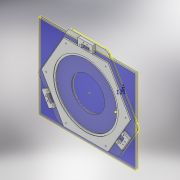
# Autodesk Inventor part: Bett Monster
Saved by Autodesk Inventor 2019 (Build 230136000, 136)
## iProperties
Created: 2018-08-03
Part Number: Bett Monster
Material: Generisch
Document SubType Name: Modeling
Designer: rene
Density: 1 g/cm^3
Appearance: Vorgabe
Author: rene
Autodesk Inventor part; units mm, degrees
ref_plane "YZ Plane" through (0, 0, 0) normal (1, 0, 0) x (0, 1, 0)
ref_plane "XZ Plane" through (0, 0, 0) normal (0, 1, 0) x (-1, 0, 0)
ref_plane "XY Plane" through (0, 0, 0) normal (0, 0, 1) x (1, 0, 0)
sketch "Bett" plane through (0, 0, 0) normal (0, 0, 1) x (1, 0, 0)
  circle A0 centre (0, 0) radius 175
  circle A1 centre (107.4996, -186.1957) radius 2.5
  line L0 (119.9996, -207.8464) -> (107.4996, -186.1957)
  line L1 (119.9996, -207.8465) -> (-120.0005, -207.8459)
  circle A2 centre (-107.5004, -186.1953) radius 2.5
  line L2 (-120.0004, -207.8459) -> (-107.5004, -186.1953)
  line L3 (-240.0001, 0.0004) -> (-120.0005, -207.8459)
  circle A3 centre (107.5004, 186.1953) radius 2.5
  line L4 (-119.9995, 207.8464) -> (120.0006, 207.8458)
  circle A4 centre (215.0001, -0.0004) radius 2.5
  line L5 (120.0006, 207.8458) -> (240.0001, -0.0006)
  circle A5 centre (-215.0001, 0.0004) radius 2.5
  line L6 (-240.0001, 0.0004) -> (-215.0001, 0.0004)
  circle A6 centre (-107.4996, 186.1957) radius 2.5
  line L7 (-240.0001, 0.0004) -> (-119.9995, 207.8464)
  line L8 (240.0001, -0.0006) -> (119.9996, -207.8465)
  circle A7 centre (0, 0) radius 165
  dimension "d0" = 350
  dimension "d1" = 240
  dimension "d2" = 207.8462
  dimension "d3" = 207.8462
  dimension "d4" = 119.9995
  dimension "d5" = 25
  dimension "d6" = 5
  dimension "d7" = 25
  dimension "d8" = 5
  dimension "d9" = 25
  dimension "d10" = 5
  dimension "d11" = 5
  dimension "d12" = 5
  dimension "d13" = 5
  dimension "d14" = 330
  constraints: 18 end point, 8 centre point, 8 coincident, 1 horizontal
  measures "d0" diameter of A0
  measures "d1" distance of L7.start L1.end
  measures "d2" distance from line of point (0, 0) L3
  measures "d3" distance from line of point (0, 0) L5
  measures "d4" horizontal distance of L5.start L5.end
  measures "d5" distance of L7.start L6.end
  measures "d6" diameter of A5
  measures "d7" distance of L0.start L0.end
  measures "d8" diameter of A1
  measures "d9" distance of L2.start L2.end
  measures "d10" diameter of A2
  measures "d11" diameter of A4
  measures "d12" diameter of A3
  measures "d13" diameter of A6
  measures "d14" diameter of A7
extrude "Extrusion Bett" add sketch "Bett" against normal blind 6 contours L1 L3 L7 L4 L5 L8
ref_plane "Arbeitsebene1" through (0, 0, -6) normal (0, 0, -1) x (-1, 0, 0)
sketch "Bett Ring" plane through (0, 0, -6) normal (0, 0, -1) x (-1, 0, 0)
  circle A0 centre (0, 0) radius 165
  circle A1 centre (0, 0) radius 175
  dimension "d18" = 350
  dimension "d19" = 330
  constraints: 2 centre point, 2 coincident
  measures "d18" diameter of A1
  measures "d19" diameter of A0
extrude "Extrusion Bett Ring" add sketch "Bett Ring" against normal blind 4
ref_plane "Arbeitsebene2" through (0, 0, -12) normal (0, 0, -1) x (-1, 0, 0)
sketch "Füsse" plane through (0, 0, -12) normal (0, 0, -1) x (-1, 0, 0)
  circle A0 centre (-107.4996, 186.1957) radius 2.5
  circle A1 centre (-107.4996, 186.1957) radius 5
  circle A2 centre (107.5004, 186.1953) radius 2.5
  circle A3 centre (107.5004, 186.1953) radius 5
  circle A4 centre (215.0001, -0.0004) radius 2.5
  circle A5 centre (215.0001, -0.0004) radius 5
  circle A6 centre (-215.0001, 0.0004) radius 5
  circle A7 centre (107.4996, -186.1957) radius 2.5
  circle A8 centre (107.4996, -186.1957) radius 5
  circle A9 centre (-107.5004, -186.1953) radius 5
  circle A10 centre (-107.5004, -186.1953) radius 2.5
  line L0 (-240.0001, 0.0004) -> (-215.0001, 0.0004)
  circle A11 centre (-215.0001, 0.0004) radius 2.5
  point P0 (0, 0)
  point P1 (0, 0)
  point P2 (0, 0)
  point P3 (0, 0)
  point P4 (0, 0)
  point P5 (0, 0)
  point P6 (0, 0)
  point P7 (165, -216.5064)
  point P8 (-165, -216.5064)
  point P9 (0, 0)
  point P10 (0, 0)
  point P11 (0, 0)
  point P12 (0, 0)
  point P13 (0, 0)
  dimension "d42" = 5
  dimension "d24" = 5
  dimension "d25" = 5
  dimension "d26" = 5
  dimension "d27" = 5
  dimension "d28" = 5
  dimension "d29" = 5
  dimension "d30" = 10
  dimension "d31" = 10
  dimension "d32" = 10
  dimension "d33" = 10
  dimension "d34" = 10
  dimension "d35" = 10
  constraints: 16 coincident, 12 centre point, 2 end point, 1 horizontal
  measures "d24" diameter of A11
  measures "d25" diameter of A7
  measures "d26" diameter of A10
  measures "d27" diameter of A4
  measures "d28" diameter of A2
  measures "d29" diameter of A0
  measures "d30" diameter of A3
  measures "d31" diameter of A5
  measures "d32" diameter of A8
  measures "d33" diameter of A9
  measures "d34" diameter of A1
  measures "d35" diameter of A6
extrude "Extrusion3" add sketch "Füsse" against normal blind 6
ref_plane "Arbeitsebene3" through (0, 0, -21) normal (0, 0, -1) x (-1, 0, 0)
sketch "Bodenplatte" plane through (0, 0, -21) normal (0, 0, -1) x (-1, 0, 0)
  circle A0 centre (-161.25, 93.0978) radius 3
  line L0 (-107.4998, 186.1959) -> (-214.9999, 0.0003) construction
  line L1 (0, 0) -> (-220.0773, 127.0617) construction
  line L2 (-262.7831, -22.1411) -> (-112.217, 238.6473)
  line L3 (-105.0001, 251.1473) -> (165, -216.5064) construction
  line L4 (-165, -216.5064) -> (104.9999, 251.1473) construction
  circle A1 centre (0, 0) radius 90
  circle A2 centre (-214.9999, 0.0003) radius 2.5
  circle A3 centre (-107.4998, 186.1959) radius 2.5
  circle A4 centre (-0.0001, 211.1473) radius 3
  line L5 (-90.5663, 251.1473) -> (90.5662, 251.1473)
  arc A5 (112.2168, 238.6473) -> (90.5662, 251.1473) centre (90.5662, 226.1473) ccw
  circle A6 centre (0, -186.1955) radius 3
  line L6 (150.5662, -216.5064) -> (-150.5663, -216.5064)
  line L7 (-270, -34.6411) -> (269.9999, -34.6411) construction
  circle A7 centre (107.4996, -186.1957) radius 2.5
  arc A8 (150.5662, -216.5064) -> (172.2168, -204.0064) centre (150.5662, -191.5064) ccw
  circle A9 centre (182.8589, -105.5736) radius 3
  line L8 (172.2168, -204.0064) -> (262.783, -47.1411)
  arc A10 (-90.5663, 251.1473) -> (-112.217, 238.6473) centre (-90.5663, 226.1473) ccw
  circle A11 centre (215.0001, -0.0004) radius 2.5
  line L9 (112.2168, 238.6473) -> (262.783, -22.1411)
  circle A12 centre (107.5004, 186.1953) radius 2.5
  circle A13 centre (161.25, 93.0978) radius 3
  line L10 (0, 0) -> (254.1234, 0) construction
  line L11 (107.5004, 186.1953) -> (215.0001, -0.0004) construction
  arc A14 (262.783, -47.1411) -> (262.783, -22.1411) centre (241.1324, -34.6411) ccw
  circle A15 centre (-107.5004, -186.1953) radius 2.5
  arc A16 (-172.2169, -204.0064) -> (-150.5663, -216.5064) centre (-150.5663, -191.5064) ccw
  circle A17 centre (-182.8589, -105.5737) radius 3
  line L12 (-172.2169, -204.0064) -> (-262.7831, -47.1411)
  arc A18 (-262.7831, -22.1411) -> (-262.7831, -47.1411) centre (-241.1325, -34.6411) ccw
  line L13 (-290, 0) -> (-289.695, 0.5283)
  dimension "d39" = 210
  dimension "d40" = 330
  dimension "d41" = 180
  dimension "d42" = 5
  dimension "d43" = 5
  dimension "d44" = 5
  dimension "d45" = 5
  dimension "d46" = 5
  dimension "d47" = 6
  dimension "d48" = 6
  dimension "d49" = 6
  dimension "d50" = 150
  dimension "d51" = 6
  dimension "d52" = 6
  dimension "d53" = 6
  dimension "d54" = 5
  constraints: 28 end point, 19 centre point, 12 point on circle, 12 tangent, 10 coincident, 3 parallel, 2 horizontal, 1 equal length, 1 perpendicular, 1 point on line
  measures "d39" distance of L3.start L4.end
  measures "d40" distance of L3.end L4.start
  measures "d41" diameter of A1
  measures "d42" diameter of A2
  measures "d43" diameter of A7
  measures "d44" diameter of A15
  measures "d45" diameter of A11
  measures "d46" diameter of A12
  measures "d47" diameter of A4
  measures "d48" diameter of A17
  measures "d49" diameter of A9
  measures "d50" angle of L10 L1
  measures "d51" diameter of A6
  measures "d52" diameter of A0
  measures "d53" diameter of A13
  measures "d54" diameter of A3
extrude "Extrusion4" add sketch "Bodenplatte" against normal blind 9
sketch "Skizze5" plane through (0, 0, -12) normal (0, 0, -1) x (-1, 0, 0)
  line L0 (0.0004, 251.1474) -> (0.0004, 250.619)
  line L1 (0.0004, 250.619) -> (0.0004, 251.1474)
  line L2 (0.0004, 250.619) -> (0.0004, 251.1474)
  line L3 (0, 231.1474) -> (20.0002, 251.1474) construction
  line L4 (0, 231.1474) -> (20.0004, 231.1478)
  line L5 (20.0004, 231.1478) -> (0.0004, 251.1471) construction
  line L6 (40.0005, 211.1469) -> (40.0005, 251.1474)
  line L7 (-172.8592, -122.8938) -> (-190.1797, -132.8938)
  circle A0 centre (-176.5195, -136.554) radius 2.6
  line L8 (-172.8592, -122.8938) -> (-180.1797, -150.2143) construction
  line L9 (-162.8592, -140.2143) -> (-172.8592, -122.8938)
  line L10 (-162.8592, -140.2143) -> (-190.1797, -132.8938) construction
  line L11 (-197.5002, -160.2143) -> (-162.8592, -140.2143)
  line L12 (-210.1801, -98.2531) -> (-192.8588, -88.2526)
  circle A1 centre (-206.5195, -84.5926) radius 2.6
  line L13 (-202.8588, -70.932) -> (-192.8588, -88.2526)
  line L14 (-192.8588, -88.2526) -> (-220.1788, -80.9317) construction
  line L15 (-202.8588, -70.932) -> (-210.1801, -98.2531) construction
  line L16 (-202.8588, -70.932) -> (-237.5002, -90.9322)
  circle A2 centre (-204.2437, -129.1252) radius 2.6
  line L17 (-190.1797, -132.8938) -> (-200.1795, -115.5737)
  line L18 (-190.1797, -132.8938) -> (-217.5, -125.5732) construction
  line L19 (-200.1795, -115.5737) -> (-208.0747, -141.8989) construction
  line L20 (-217.5002, -125.5733) -> (-217.0427, -125.3091)
  line L21 (-217.0427, -125.3091) -> (-217.5002, -125.5733)
  line L22 (-217.0427, -125.3091) -> (-217.5002, -125.5733)
  circle A3 centre (-213.8398, -111.9133) radius 2.6
  line L23 (-237.5002, -90.9322) -> (-197.5002, -160.2143)
  line L24 (-200.1795, -115.5737) -> (-210.1801, -98.2531)
  line L25 (-210.1801, -98.2531) -> (-217.5, -125.5732) construction
  line L26 (-200.1795, -115.5737) -> (-227.5001, -108.253) construction
  line L27 (162.8584, -140.2149) -> (172.8584, -122.8943)
  line L28 (190.1797, -132.8947) -> (172.8584, -122.8943)
  circle A4 centre (176.519, -136.5548) radius 2.6
  line L29 (172.8584, -122.8943) -> (180.1783, -150.2146) construction
  line L30 (162.8584, -140.2149) -> (190.1797, -132.8947) construction
  line L31 (162.8584, -140.2149) -> (197.4998, -160.2151)
  circle A5 centre (203.8397, -129.234) radius 2.6
  line L32 (200.1795, -115.5737) -> (190.1797, -132.8947)
  line L33 (182.8584, -105.5739) -> (182.8586, -105.5735)
  line L34 (182.8586, -105.5735) -> (182.8584, -105.5739)
  line L35 (190.1797, -132.8947) -> (217.4995, -125.5739) construction
  line L36 (200.1795, -115.5737) -> (207.4999, -142.8944) construction
  line L37 (217.0422, -125.3099) -> (217.4998, -125.5741)
  line L38 (217.4998, -125.5741) -> (217.0422, -125.3099)
  line L39 (217.0422, -125.3099) -> (217.4998, -125.5741)
  circle A6 centre (213.9476, -112.3176) radius 2.6
  line L40 (197.4998, -160.2151) -> (237.4998, -90.9331)
  line L41 (210.1792, -98.2536) -> (200.1795, -115.5737)
  line L42 (210.1792, -98.2536) -> (217.4995, -125.5739) construction
  line L43 (200.1795, -115.5737) -> (226.9253, -109.2485) construction
  line L44 (192.8587, -88.2536) -> (210.1792, -98.2536)
  circle A7 centre (206.519, -84.5933) radius 2.6
  line L45 (192.8587, -88.2536) -> (220.1792, -80.9331) construction
  line L46 (202.8587, -70.9331) -> (192.8587, -88.2536)
  line L47 (237.4998, -90.9331) -> (202.8587, -70.9331)
  line L48 (202.8587, -70.9331) -> (210.1792, -98.2536) construction
  line L49 (0, 211.1469) -> (0.0005, 211.1469)
  line L50 (0.0005, 211.1469) -> (0, 211.1469)
  line L51 (-182.8586, -105.5735) -> (-182.8588, -105.573)
  circle A8 centre (-29.9995, 221.1474) radius 2.6
  line L52 (-19.9995, 211.1474) -> (-39.9995, 231.1474) construction
  line L53 (-182.8588, -105.573) -> (-182.8586, -105.5735)
  line L54 (40.0005, 211.1469) -> (20.0004, 211.1469)
  circle A9 centre (30.0004, 221.1474) radius 2.6
  line L55 (20.0004, 211.1469) -> (40.0005, 231.1463) construction
  line L56 (40.0005, 211.1469) -> (20.0004, 231.1478) construction
  circle A10 centre (10.0001, 241.1474) radius 2.6
  line L57 (20.0004, 231.1478) -> (20.0004, 211.1469)
  line L58 (40.0005, 251.1474) -> (-39.9995, 251.1474)
  circle A11 centre (-9.7039, 241.4429) radius 2.6
  line L59 (0, 231.1474) -> (-18.8507, 251.1474) construction
  line L60 (-19.9995, 231.1474) -> (0, 231.1474)
  line L61 (-19.9995, 211.1474) -> (-19.9995, 231.1474)
  line L62 (-39.9995, 211.1474) -> (-19.9995, 211.1474)
  line L63 (-39.9995, 211.1474) -> (-19.9995, 231.1474) construction
  line L64 (-39.9995, 251.1474) -> (-39.9995, 211.1474)
  line L65 (-19.9995, 231.1474) -> (0.0004, 251.1471) construction
  point P0 (0, 0)
  point P1 (0, 0)
  point P2 (0, 0)
  point P3 (0, 0)
  dimension "d57" = 40
  dimension "d58" = 40
  dimension "d59" = 80
  dimension "d60" = 20
  dimension "d61" = 5.2
  dimension "d62" = 5.2
  dimension "d63" = 5.2
  dimension "d64" = 5.2
  dimension "d65" = 40
  dimension "d66" = 40
  dimension "d67" = 80
  dimension "d68" = 20
  dimension "d69" = 5.2
  dimension "d70" = 5.2
  dimension "d71" = 5.2
  dimension "d72" = 5.2
  dimension "d73" = 40
  dimension "d74" = 40
  dimension "d75" = 80
  dimension "d76" = 20
  dimension "d77" = 5.2
  dimension "d78" = 5.2
  dimension "d79" = 5.2
  dimension "d80" = 5.2
  constraints: 132 end point, 15 parallel, 12 centre point, 12 midpoint, 12 point on line, 6 perpendicular, 3 collinear
  measures "d57" distance of L9.start L11.start
  measures "d58" distance of L15.start L51.end
  measures "d59" distance between parallel lines of L11 L16
  measures "d60" distance between parallel lines of L11 L7
  measures "d61" diameter of A2
  measures "d62" diameter of A3
  measures "d63" diameter of A0
  measures "d64" diameter of A1
  measures "d65" distance of L46.start L40.end
  measures "d66" distance of L27.start L33.start
  measures "d67" distance between parallel lines of L47 L31
  measures "d68" distance between parallel lines of L47 L44
  measures "d69" diameter of A6
  measures "d70" diameter of A5
  measures "d71" diameter of A7
  measures "d72" diameter of A4
  measures "d73" distance of L63.start L58.end
  measures "d74" distance of L6.start L49.end
  measures "d75" distance between parallel lines of L64 L6
  measures "d76" distance between parallel lines of L64 L61
  measures "d77" diameter of A11
  measures "d78" diameter of A10
  measures "d79" diameter of A8
  measures "d80" diameter of A9
extrude "Extrusion6" add sketch "Skizze5" against normal blind 15
sketch "Gummifüsse" plane through (0, 0, -21) normal (0, 0, -1) x (-1, 0, 0)
  circle A0 centre (0, 0) radius 90 projected
  circle A1 centre (-182.8589, -105.5737) radius 3 projected
  circle A2 centre (182.8589, -105.5736) radius 3 projected
  circle A3 centre (0, -186.1955) radius 3 projected
  circle A4 centre (161.25, 93.0978) radius 3 projected
  circle A5 centre (-0.0001, 211.1473) radius 3 projected
  circle A6 centre (-161.25, 93.0978) radius 3 projected
  circle A7 centre (-214.9999, 0.0003) radius 2.5 projected
  circle A8 centre (-107.4998, 186.1959) radius 2.5 projected
  arc A9 (-262.7831, -22.1411) -> (-262.7831, -47.1411) centre (-241.1325, -34.6411) ccw projected
  line L0 (-262.7831, -22.1411) -> (-112.217, 238.6473) projected
  arc A10 (-90.5663, 251.1473) -> (-112.217, 238.6473) centre (-90.5663, 226.1473) ccw projected
  line L1 (-90.5663, 251.1473) -> (90.5662, 251.1473) projected
  arc A11 (112.2168, 238.6473) -> (90.5662, 251.1473) centre (90.5662, 226.1473) ccw projected
  line L2 (112.2168, 238.6473) -> (262.783, -22.1411) projected
  arc A12 (262.783, -47.1411) -> (262.783, -22.1411) centre (241.1324, -34.6411) ccw projected
  line L3 (262.783, -47.1411) -> (172.2168, -204.0064) projected
  arc A13 (150.5662, -216.5064) -> (172.2168, -204.0064) centre (150.5662, -191.5064) ccw projected
  line L4 (150.5662, -216.5064) -> (-150.5663, -216.5064) projected
  arc A14 (-172.2169, -204.0064) -> (-150.5663, -216.5064) centre (-150.5663, -191.5064) ccw projected
  line L5 (-172.2169, -204.0064) -> (-262.7831, -47.1411) projected
  circle A15 centre (-107.5004, -186.1953) radius 2.5 projected
  circle A16 centre (215.0001, -0.0004) radius 2.5 projected
  circle A17 centre (107.5004, 186.1953) radius 2.5 projected
  circle A18 centre (107.4996, -186.1957) radius 2.5 projected
ref_plane "Arbeitsebene4" through (161.25, 93.0978, -21) normal (-1, 0.0000001, 0) x (-0.0000001, -1, 0)
ref_plane "Arbeitsebene5" through (0.0001, 211.1473, -21) normal (-1, 0.0000001, 0) x (-0.0000001, -1, 0)
ref_plane "Arbeitsebene6" through (-161.25, 93.0978, -21) normal (-1, 0.0000001, 0) x (-0.0000001, -1, 0)
ref_plane "Arbeitsebene7" through (-182.8589, -105.5736, -21) normal (-1, 0.0000001, 0) x (-0.0000001, -1, 0)
ref_plane "Arbeitsebene8" through (0, -186.1955, -21) normal (-1, 0.0000001, 0) x (-0.0000001, -1, 0)
ref_plane "Arbeitsebene9" through (182.8589, -105.5737, -21) normal (-1, 0.0000001, 0) x (-0.0000001, -1, 0)
sketch "Skizze7" plane through (161.25, 93.0978, -21) normal (-1, 0.0000001, 0) x (-0.0000001, -1, 0)
  line L0 (0, 12.5064) -> (0, -26.7472)
  line L1 (3, 0) -> (3, -14)
  line L2 (5, -14) -> (5, -20)
  line L3 (5, -14) -> (3, -14)
  line L4 (3, 0) -> (15, 0)
  line L5 (5, -20) -> (9.2192, -20)
  line L6 (10.1894, -19.2425) -> (15, 0)
  arc A0 (9.2192, -20) -> (10.1894, -19.2425) centre (9.2192, -19) ccw
  point P0 (93.0978, 21)
  point P1 (10, -20)
  dimension "d135" = 12
  dimension "d136" = 5
  dimension "d137" = 1
  constraints: 14 end point, 3 vertical, 2 horizontal, 2 point on circle, 2 point on line, 2 tangent, 1 centre point, 1 perpendicular
  measures "d135" distance of L1.start L4.end
  measures "d136" distance of L2.end point (10, -20)
  measures "d137" radius of A0
sketch "Skizze10" plane through (0.0001, 211.1473, -21) normal (-1, 0.0000001, 0) x (-0.0000001, -1, 0)
  line L0 (0, 12.5064) -> (0, -26.7472)
  line L1 (3, 0) -> (3, -14)
  line L2 (5, -14) -> (5, -20)
  line L3 (5, -14) -> (3, -14)
  line L4 (3, 0) -> (15, 0)
  line L5 (5, -20) -> (9.2192, -20)
  line L6 (10.1894, -19.2425) -> (15, 0)
  arc A0 (9.2192, -20) -> (10.1894, -19.2425) centre (9.2192, -19) ccw
  point P0 (211.1473, 21)
  point P1 (10, -20)
  dimension "d139" = 12
  dimension "d140" = 5
  dimension "d141" = 1
  constraints: 14 end point, 3 vertical, 2 horizontal, 2 point on circle, 2 point on line, 2 tangent, 1 centre point, 1 perpendicular
  measures "d139" distance of L1.start L4.end
  measures "d140" distance of L2.end point (10, -20)
  measures "d141" radius of A0
sketch "Skizze11" plane through (-161.25, 93.0978, -21) normal (-1, 0.0000001, 0) x (-0.0000001, -1, 0)
  line L0 (0, 12.5064) -> (0, -26.7472)
  line L1 (3, 0) -> (3, -14)
  line L2 (5, -14) -> (5, -20)
  line L3 (5, -14) -> (3, -14)
  line L4 (3, 0) -> (15, 0)
  line L5 (5, -20) -> (9.2192, -20)
  line L6 (10.1894, -19.2425) -> (15, 0)
  arc A0 (9.2192, -20) -> (10.1894, -19.2425) centre (9.2192, -19) ccw
  point P0 (93.0977, 21)
  point P1 (10, -20)
  dimension "d142" = 12
  dimension "d143" = 5
  dimension "d144" = 1
  constraints: 14 end point, 3 vertical, 2 horizontal, 2 point on circle, 2 point on line, 2 tangent, 1 centre point, 1 perpendicular
  measures "d142" distance of L1.start L4.end
  measures "d143" distance of L2.end point (10, -20)
  measures "d144" radius of A0
sketch "Skizze12" plane through (-182.8589, -105.5736, -21) normal (-1, 0.0000001, 0) x (-0.0000001, -1, 0)
  line L0 (0, 12.5064) -> (0, -26.7472)
  line L1 (3, 0) -> (3, -14)
  line L2 (5, -14) -> (5, -20)
  line L3 (5, -14) -> (3, -14)
  line L4 (3, 0) -> (15, 0)
  line L5 (5, -20) -> (9.2192, -20)
  line L6 (10.1894, -19.2425) -> (15, 0)
  arc A0 (9.2192, -20) -> (10.1894, -19.2425) centre (9.2192, -19) ccw
  point P0 (-105.5736, 21)
  point P1 (10, -20)
  dimension "d145" = 12
  dimension "d146" = 5
  dimension "d147" = 1
  constraints: 14 end point, 3 vertical, 2 horizontal, 2 point on circle, 2 point on line, 2 tangent, 1 centre point, 1 perpendicular
  measures "d145" distance of L1.start L4.end
  measures "d146" distance of L2.end point (10, -20)
  measures "d147" radius of A0
sketch "Skizze13" plane through (0, -186.1955, -21) normal (-1, 0.0000001, 0) x (-0.0000001, -1, 0)
  line L0 (0, 12.5064) -> (0, -26.7472)
  line L1 (0, 12.5064) -> (0, -26.7472)
  line L2 (0, 12.5064) -> (0, -26.7472)
  line L3 (3, 0) -> (3, -14)
  line L4 (5, -14) -> (5, -20)
  line L5 (5, -14) -> (3, -14)
  line L6 (3, 0) -> (15, 0)
  line L7 (5, -20) -> (9.2192, -20)
  line L8 (10.1894, -19.2425) -> (15, 0)
  arc A0 (9.2192, -20) -> (10.1894, -19.2425) centre (9.2192, -19) ccw
  point P0 (-186.1955, 21)
  point P1 (10, -20)
  dimension "d158" = 12
  dimension "d159" = 5
  dimension "d160" = 1
  constraints: 18 end point, 5 vertical, 2 horizontal, 2 point on circle, 2 point on line, 2 tangent, 1 centre point, 1 perpendicular
  measures "d158" distance of L3.start L6.end
  measures "d159" distance of L4.end point (10, -20)
  measures "d160" radius of A0
sketch "Skizze14" plane through (182.8589, -105.5737, -21) normal (-1, 0.0000001, 0) x (-0.0000001, -1, 0)
  line L0 (0, 12.5064) -> (0, -26.7472)
  line L1 (3, 0) -> (3, -14)
  line L2 (5, -14) -> (5, -20)
  line L3 (5, -14) -> (3, -14)
  line L4 (3, 0) -> (15, 0)
  line L5 (5, -20) -> (9.2192, -20)
  line L6 (10.1894, -19.2425) -> (15, 0)
  arc A0 (9.2192, -20) -> (10.1894, -19.2425) centre (9.2192, -19) ccw
  point P0 (-105.5737, 21)
  point P1 (10, -20)
  dimension "d151" = 12
  dimension "d152" = 5
  dimension "d153" = 1
  constraints: 14 end point, 3 vertical, 2 horizontal, 2 point on circle, 2 point on line, 2 tangent, 1 centre point, 1 perpendicular
  measures "d151" distance of L1.start L4.end
  measures "d152" distance of L2.end point (10, -20)
  measures "d153" radius of A0
revolve "Umdrehung7" add sketch "Skizze7" angle 360 about axis through (161.25, 93.0978, -8.4936) along (0, 0, -1)
revolve "Umdrehung8" add sketch "Skizze10" angle 360 about axis through (0.0001, 211.1473, -8.4936) along (0, 0, -1)
revolve "Umdrehung9" add sketch "Skizze14" angle 360 about axis through (182.8589, -105.5737, -8.4936) along (0, 0, -1)
revolve "Umdrehung10" add sketch "Skizze11" angle 360 about axis through (-161.25, 93.0978, -8.4936) along (0, 0, -1)
revolve "Umdrehung11" add sketch "Skizze12" angle 360 about axis through (-182.8589, -105.5736, -8.4936) along (0, 0, -1)
revolve "Umdrehung12" add sketch "Skizze13" angle 360 about axis through (0, -186.1955, -8.4936) along (0, 0, -1)
